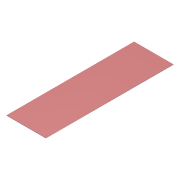
# Autodesk Inventor part: HousingCage_Sidepanel_long
Saved by Autodesk Inventor 2016 (Build 200138000, 138)
## iProperties
Created: 2012-11-26
Part Number: HousingCage_Sidepanel_long
Material: PMMA Plastic
Document SubType Name: Modeling
Designer: Neef
Mass: 347.49 g
Surface Area: 1998 cm^2
Volume: 292.5 cm^3
Density: 1.188 g/cm^3
Appearance: Dark Red
Author: Neef
Autodesk Inventor part; units mm, degrees
ref_plane "YZ Plane" through (0, 0, 0) normal (1, 0, 0) x (0, 1, 0)
ref_plane "XZ Plane" through (0, 0, 0) normal (0, 1, 0) x (-1, 0, 0)
ref_plane "XY Plane" through (0, 0, 0) normal (0, 0, 1) x (1, 0, 0)
sketch "Skizze1" plane through (0, 0, 0) normal (0, 0, 1) x (1, 0, 0)
  line L0 (-100, 325) -> (100, 325)
  line L1 (100, 325) -> (100, -325)
  line L2 (100, -325) -> (-100, -325)
  line L3 (-100, -325) -> (-100, 325)
  line L4 (0, 455) -> (0, -455) projected
  line L5 (-140, 0) -> (140, 0) projected
  point P0 (0, 0)
  point P1 (0, 325)
  point P2 (100, 0)
  dimension "d0" = 200
  dimension "d1" = 650
  constraints: 8 end point, 2 midpoint, 2 parallel, 2 point on line, 1 horizontal, 1 perpendicular
  measures "d0" distance of L0.start L0.end
  measures "d1" distance of L2.end L0.start
extrude "Extrusion1" add sketch "Skizze1" along normal blind 3
